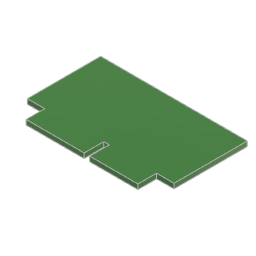
TinyTendo Cartridge-Shell (Autodesk Fusion 360 archive; units mm, degrees)
design "TinyTendo NROM PCB"
Autodesk Fusion 360 part; units mm, degrees
sketch "Sketch1" plane through (0, 0, 0) normal (0, 0, 1) x (1, 0, 0)
  line L0 (24, -15.05) -> (-24, -15.05)
  line L1 (-24, -15.05) -> (-24, 15.05)
  line L2 (-24, 15.05) -> (24, 15.05)
  line L3 (24, 15.05) -> (24, -15.05)
  line L4 (24, -15.05) -> (-24, 15.05) construction
  line L5 (-24, -15.05) -> (24, 15.05) construction
  line L6 (24, -15.05) -> (18.3, -15.05)
  line L7 (18.3, -15.05) -> (18.3, -8.95)
  line L8 (18.3, -8.95) -> (24, -8.95)
  line L9 (-24, -15.05) -> (-18.3, -15.05)
  line L10 (-18.3, -15.05) -> (-18.3, -8.95)
  line L11 (-18.3, -8.95) -> (-24, -8.95)
  line L12 (-18.3, -15.05) -> (0.7, -15.05)
  line L13 (18.3, -15.05) -> (2.5, -15.05)
  line L14 (2.5, -15.05) -> (2.5, -8.65)
  line L15 (2.5, -8.65) -> (0.7, -8.65)
  line L16 (0.7, -8.65) -> (0.7, -15.05)
  dimension "d1" = 48
  dimension "d2" = 30.1
  dimension "d3" = 5.7
  dimension "d4" = 6.1
  dimension "d5" = 5.7
  dimension "d6" = 6.1
  dimension "d7" = 19
  dimension "d8" = 15.8
  dimension "d9" = 6.4
  constraint horizontal L0
  constraint perpendicular L0 L1
  constraint parallel L0 L2
  constraint parallel L1 L3
  constraint coincident L4 origin
  constraint coincident L5 origin
  constraint perpendicular L3 L6
  constraint perpendicular L6 L7
  constraint coincident L3 L8.end
  constraint perpendicular L3 L8
  constraint perpendicular L1 L9
  constraint perpendicular L9 L10
  constraint coincident L1 L11.end
  constraint perpendicular L1 L11
  constraint perpendicular L10 L12
  constraint perpendicular L7 L13
  constraint perpendicular L13 L14
  constraint perpendicular L14 L15
  constraint perpendicular L0 L16
  measures "d1" distance of L1.end L2.end
  measures "d2" distance of L0.end L1.end
  measures "d3" distance of L0.start L6.end
  measures "d4" distance of L6.end L7.end
  measures "d5" distance of L0.end L9.end
  measures "d6" distance of L9.end L10.end
  measures "d7" distance of L9.end L12.end
  measures "d8" distance of L6.end L13.end
  measures "d9" distance of L13.end L14.end
extrude "Extrude1" add sketch "Sketch1" along normal blind 1.6 contours L0 L1 L2 L3 L7 L8 L10 L11 L12 L13 L14 L15 L16
